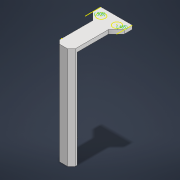
# Autodesk Inventor part: Vertical Beam Prototype
Saved by Autodesk Inventor 2022 (Build 260153000, 153)
## iProperties
Created: 2021-05-30
Part Number: Vertical Beam Prototype
Material: Generic
Document SubType Name: Modeling
Designer: sidsa
Density: 1 g/cm^3
Appearance: Default
Author: sidsa
## iProperties of the stored document Vertical Beam Prototype_3DPrint.ipt
Created: 2021-05-30
Part Number: Vertical Beam Prototype_3DPrint
Material: Generic
Document SubType Name: Modeling
Designer: sidsa
Density: 1 g/cm^3
Appearance: Default
Author: sidsa
Autodesk Inventor part; units mm, degrees
ref_plane "YZ Plane" through (0, 0, 0) normal (1, 0, 0) x (0, 1, 0)
ref_plane "XZ Plane" through (0, 0, 0) normal (0, 1, 0) x (-1, 0, 0)
ref_plane "XY Plane" through (0, 0, 0) normal (0, 0, 1) x (1, 0, 0)
sketch "Sketch1" plane through (0, 0, 0) normal (0, 0, 1) x (1, 0, 0)
  line L0 (0, 0) -> (25.4, 0)
  line L1 (25.4, 0) -> (25.4, 165.1)
  line L2 (25.4, 165.1) -> (0, 165.1)
  line L3 (0, 165.1) -> (0, 0)
  line L4 (16.2837, 38.7604) -> (19.9133, 32.4739)
  line L5 (19.9133, 32.4739) -> (16.2837, 26.1874)
  line L6 (16.2837, 26.1874) -> (9.0247, 26.1874)
  line L7 (9.0247, 26.1874) -> (5.3952, 32.4739)
  line L8 (5.3952, 32.4739) -> (9.0247, 38.7604)
  line L9 (9.0247, 38.7604) -> (16.2837, 38.7604)
  line L10 (12.7, 0) -> (12.6542, 32.4739)
  dimension "d0" = 25.4
  dimension "d1" = 165.1
  dimension "d2" = 12.573
  dimension "d3" = 26.1874
  constraints: 22 end point, 3 parallel, 1 horizontal, 1 midpoint, 1 perpendicular, 13 other
  measures "d0" distance of L1.end L2.end
  measures "d1" distance of L0.end L1.end
  measures "d2" distance between parallel lines of L6 L9
  measures "d3" distance between parallel lines of L0 L6
extrude "Extrusion1" add sketch "Sketch1" along normal blind 3.175
sketch "Sketch2" plane through (0, 0, 0) normal (0, 0, -1) x (-1, 0, 0)
  line L0 (-25.4, 0) -> (-25.4, 165.1) projected
  line L1 (0, 0) -> (-25.4, 0) projected
  line L2 (0, 165.1) -> (0, 0) projected
  line L3 (-25.4, 165.1) -> (0, 165.1) projected
  line L4 (-16.2837, 26.1874) -> (-9.0247, 26.1874) projected
  line L5 (-19.9133, 32.4739) -> (-16.2837, 26.1874) projected
  line L6 (-16.2837, 38.7604) -> (-19.9133, 32.4739) projected
  line L7 (-9.0247, 38.7604) -> (-16.2837, 38.7604) projected
  line L8 (-5.3952, 32.4739) -> (-9.0247, 38.7604) projected
  line L9 (-9.0247, 26.1874) -> (-5.3952, 32.4739) projected
  line L10 (-16.2984, 26.035) -> (-19.9646, 32.385) projected
  line L11 (-5.2999, 32.385) -> (-8.9661, 26.035) projected
  line L12 (-8.9661, 26.035) -> (-16.2984, 26.035) projected
  line L13 (-16.2984, 26.035) -> (-19.9646, 32.385) projected
  line L14 (-19.9646, 32.385) -> (-16.2984, 38.735) projected
  line L15 (-16.2984, 38.735) -> (-8.9661, 38.735) projected
  line L16 (-8.9661, 38.735) -> (-5.2999, 32.385) projected
  line L17 (-41.2072, 1.27) -> (15.9428, 1.27) projected
  line L18 (15.9428, 1.27) -> (15.9428, 63.5) projected
  line L19 (-41.2072, 63.5) -> (15.9428, 63.5) projected
  line L20 (-41.2072, 1.27) -> (-41.2072, 63.5) projected
  dimension "d32" = 12.573
  dimension "d33" = 12.7
  measures "d32" distance between parallel lines of L7 L4
  measures "d33" distance between parallel lines of L12 L15
extrude "Extrusion2" add sketch "Sketch2" along normal blind 6.35 and the other way blind 3.175 contours L5 L6 L15 L8 L9 L4 | L6 L7 L8 L15
sketch "Sketch3" plane through (0, 0, 3.175) normal (0, 0, 1) x (1, 0, 0)
  line L0 (25.4, 0) -> (25.4, 165.1) projected
  line L1 (25.4, 165.1) -> (0, 165.1) projected
  line L2 (0, 165.1) -> (0, 0) projected
  line L3 (0, 0) -> (25.4, 0) projected
extrude "Extrusion3" add sketch "Sketch3" along normal blind 6.35
chamfer "Chamfer1" distance 6.35 angle 45 2 edges at (25.4, 82.55, 9.525) (0, 82.55, 9.525)
sketch "Sketch5" plane through (9.0247, 38.7604, 0) normal (0, 1, 0) x (1, 0, 0)
  line L0 (7.259, 0) -> (7.259, 6.35) projected
  line L1 (32.1825, 2.54) -> (-24.9675, 2.54) projected
  line L2 (0, 0) -> (0, 6.35) projected
  line L3 (7.259, 0) -> (7.259, 6.35) projected
  line L4 (0, 6.35) -> (0, 0) projected
  line L5 (7.259, 2.54) -> (0, 2.54)
  line L6 (0, 2.54) -> (0, 6.35)
  line L7 (0, 6.35) -> (7.259, 6.35)
  line L8 (7.259, 6.35) -> (7.259, 2.54)
  line L9 (5.989, 3.175) -> (1.27, 3.175)
  line L10 (1.27, 3.175) -> (1.27, 5.715)
  line L11 (1.27, 5.715) -> (5.989, 5.715)
  line L12 (5.989, 5.715) -> (5.989, 3.175)
  point P0 (-9.0247, 0)
  dimension "d25" = 0.635
  dimension "d26" = 1.27
  dimension "d27" = 0.635
  dimension "d28" = 1.27
  dimension "d29" = 2.54
  constraints: 16 end point, 4 parallel, 2 horizontal, 2 perpendicular, 2 point on line
  measures "d25" distance between parallel lines of L1 L9
  measures "d26" distance between parallel lines of L2 L10
  measures "d27" distance between parallel lines of L7 L11
  measures "d28" distance between parallel lines of L0 L12
  measures "d29" distance between parallel lines of L11 L9
extrude "Extrusion5" cut sketch "Sketch5" against normal blind 12.7 contours L9 L10 L11 L12
sketch "Sketch6" plane through (0, 0, 0) normal (0, 0, -1) x (-1, 0, 0)
  line L0 (-25.4, 0) -> (-25.4, 165.1) projected
  line L1 (0, 0) -> (-25.4, 0) projected
  line L2 (0, 165.1) -> (0, 0) projected
  line L3 (-25.4, 165.1) -> (0, 165.1) projected
  line L4 (-16.2837, 26.1874) -> (-9.0247, 26.1874) projected
  line L5 (-19.9133, 32.4739) -> (-16.2837, 26.1874) projected
  line L6 (-16.2837, 38.7604) -> (-19.9133, 32.4739) projected
  line L7 (-9.0247, 38.7604) -> (-16.2837, 38.7604) projected
  line L8 (-5.3952, 32.4739) -> (-9.0247, 38.7604) projected
  line L9 (-9.0247, 26.1874) -> (-5.3952, 32.4739) projected
  line L10 (0, 165.1) -> (0, 0) projected
  line L11 (-25.4, 165.1) -> (0, 165.1)
  line L12 (0, 165.1) -> (0, 158.75)
  line L13 (0, 158.75) -> (-25.4, 158.75)
  line L14 (-25.4, 158.75) -> (-25.4, 165.1)
  point P0 (-25.4, 158.75)
  dimension "d34" = 6.35
  constraints: 8 end point, 2 parallel, 1 horizontal, 1 perpendicular, 1 point on line
  measures "d34" distance of L11.end L12.end
extrude "Extrusion6" add sketch "Sketch6" along normal blind 76.2 contours L0 L3 L2 L13
sketch "Sketch7" plane through (0, 0, 3.175) normal (-1, 0, 0) x (0, 0, 1)
  line L0 (-79.375, 165.1) -> (0, 165.1) projected
  line L1 (-3.175, 158.75) -> (-79.375, 158.75) projected
  line L2 (-79.375, 165.1) -> (-53.975, 165.1)
  line L3 (-53.975, 165.1) -> (-53.975, 158.75)
  line L4 (-53.975, 158.75) -> (-79.375, 158.75)
  line L5 (-79.375, 158.75) -> (-79.375, 165.1)
  point P0 (-3.175, 0)
  dimension "d37" = 25.4
  constraints: 8 end point, 2 parallel, 1 horizontal, 1 perpendicular, 1 point on line
  measures "d37" distance of L3.end L4.end
extrude "Extrusion7" add sketch "Sketch7" along normal blind 12.7
sketch "Sketch8" plane through (25.4, 0, 3.175) normal (1, 0, 0) x (0, 0, -1)
  line L0 (79.375, 165.1) -> (0, 165.1) projected
  line L1 (79.375, 165.1) -> (53.975, 165.1)
  line L2 (53.975, 165.1) -> (53.975, 158.75)
  line L3 (53.975, 158.75) -> (79.375, 158.75)
  line L4 (79.375, 158.75) -> (79.375, 165.1)
  point P0 (3.175, 0)
  dimension "d40" = 25.4
  dimension "d41" = 6.35
  constraints: 8 end point, 2 parallel, 1 horizontal, 1 perpendicular
  measures "d40" distance of L3.end L2.end
  measures "d41" distance of L2.end L1.end
extrude "Extrusion8" add sketch "Sketch8" along normal blind 12.7
sketch "Sketch9" plane through (6.35, 165.1, 9.525) normal (0, 1, 0) x (1, 0, 0)
  circle A0 centre (-6.2737, 72.0756) radius 6.55 projected
  circle A1 centre (19.3263, 72.0756) radius 6.55 projected
  line L0 (31.75, 85.725) -> (31.75, 60.325) projected
  line L1 (-19.05, 60.325) -> (-19.05, 85.725) projected
  line L2 (31.75, 60.325) -> (31.75, 85.725) projected
  line L3 (31.75, 71.286) -> (25.8285, 71.286)
  line L4 (12.8241, 71.286) -> (-19.05, 71.286)
  line L5 (31.75, 71.286) -> (27.2796, 71.286)
  line L6 (27.2796, 71.286) -> (19.1516, 71.286)
  circle A2 centre (19.1516, 71.286) radius 8.128
  line L7 (-19.05, 71.286) -> (-6.4516, 71.286)
  circle A3 centre (-6.4516, 71.286) radius 8.128
  point P0 (-6.35, 9.525)
  point P1 (1.6764, 71.286)
  point P2 (-14.5796, 71.286)
  point P3 (-12.7759, 71.286)
  point P4 (0.2285, 71.286)
  dimension "d49" = 25.6
  dimension "d50" = 4.4704
  dimension "d51" = 8.128
  dimension "d52" = 16.256
  dimension "d53" = 12.5984
  dimension "d54" = 16.256
  constraints: 10 end point, 5 point on line, 2 centre point, 2 coincident, 2 perpendicular, 2 point on circle
  measures "d49" distance of A0.centre A1.centre
  measures "d50" distance of L3.start L5.end
  measures "d51" distance of L5.end L6.end
  measures "d52" diameter of A2
  measures "d53" distance of L4.end L7.end
  measures "d54" diameter of A3
extrude "Extrusion9" cut sketch "Sketch9" against normal blind 6.35
chamfer "Chamfer5" distance 12.7 angle 45 2 edges at (25.4, 161.925, -50.8) (0, 161.925, -50.8)
body "Solid1"
